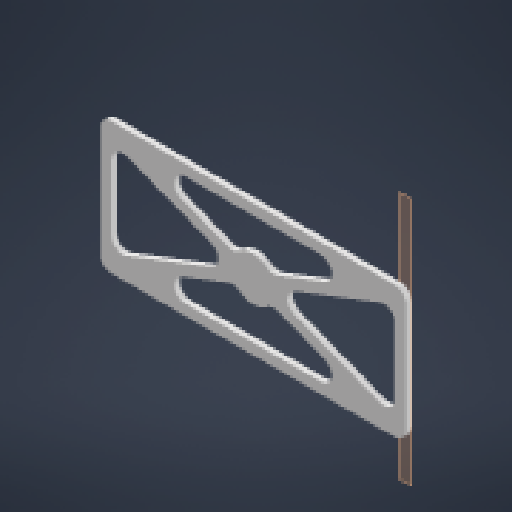
# Autodesk Inventor part: bracing
Saved by Autodesk Inventor 2026.3 (Build 303398000, 398)
## iProperties
Created: 2026-05-06
Part Number: bracing
Material: Generic
Document SubType Name: Modeling
Designer: frede
Density: 1 g/cm^3
Appearance: Default
Author: frede
Autodesk Inventor part; units mm, degrees
ref_plane "YZ Plane" through (0, 0, 0) normal (1, 0, 0) x (0, 1, 0)
ref_plane "XZ Plane" through (0, 0, 0) normal (0, 1, 0) x (-1, 0, 0)
ref_plane "XY Plane" through (0, 0, 0) normal (0, 0, 1) x (1, 0, 0)
ref_plane "Work Plane1" through (0, 0, 0) normal (0, 0, 1) x (1, 0, 0)
sketch "Sketch1" plane through (0, 0, 0) normal (0, 0, 1) x (1, 0, 0)
  line L0 (5, -30) -> (5, -90)
  line L1 (-134, -30) -> (-134, -90)
  line L2 (5, -90) -> (-134, -90)
  line L3 (-134, -30) -> (5, -30)
  line L4 (5, 0) -> (5, -102.9406) projected
  line L5 (0, -35) -> (-129, -35)
  line L6 (-129, -35) -> (-129, -85)
  line L7 (-129, -85) -> (0, -85)
  line L8 (0, -85) -> (0, -35)
  line L9 (0, -35) -> (-129, -85)
  line L10 (0, -85) -> (-129, -35)
  circle A0 centre (-64.5, -60) radius 10
  circle A1 centre (-64.5, -60) radius 2.5
  line L11 (0, -82.3188) -> (-122.0824, -35)
  line L12 (-6.9176, -85) -> (-129, -37.6812)
  line L13 (-122.0824, -85) -> (0, -37.6812)
  line L14 (-129, -82.3188) -> (-6.9176, -35)
  point P0 (0, 0)
  point P1 (-43.2477, -65.5561)
  point P2 (-40.0223, -72.1687)
  point P3 (-54.5685, -58.8318)
  point P4 (0, -17.9417)
  point P5 (-54.5685, -61.1682)
  point P6 (-74.4315, -58.8318)
  point P7 (-72.6245, -54.1697)
  point P8 (-72.6245, -65.8303)
  point P9 (-56.3755, -65.8303)
  point P10 (-57.5824, -60)
  point P11 (-74.4315, -61.1682)
  point P12 (-56.3755, -54.1697)
  dimension "d0" = 60
  dimension "d1" = 139
  dimension "d2" = 0
  dimension "d3" = 50
  dimension "d4" = 129
  dimension "d5" = 5
  dimension "d6" = 5
  dimension "d7" = 20
  dimension "d8" = 5
  dimension "d14" = 30
  constraints: 28 end point, 10 point on line, 8 parallel, 4 tangent, 2 centre point, 2 horizontal, 1 coincident, 1 midpoint, 1 perpendicular
  measures "d0" distance between parallel lines of L3 L2
  measures "d1" distance between parallel lines of L1 L0
  measures "d2" distance between parallel lines of L4 L0
  measures "d3" distance of L6.end L5.end
  measures "d4" distance between parallel lines of L6 L8
  measures "d5" distance between parallel lines of L2 L7
  measures "d6" distance between parallel lines of L0 L8
  measures "d7" diameter of A0
  measures "d8" diameter of A1
  measures "d14" distance from line of point (0, 0) L3
extrude "Extrusion1" add sketch "Sketch1" along normal blind 2.5 contours L0 L2 L1 L3 | L9 A0 L14 L5 | L8 L13 A0 L9 | A0 L13 L11 L9 | L9 L11 L14 A0 | L11 A0 L10 L5 | L14 L11 A0 | L8 L10 A0 L11 | A0 L11 L13 | L11 L13 L10 A1 L9 | L9 A1 L11 | L10 A0 L12 L6 | L11 L14 L10 A0 | L11 A1 L14 | L7 L12 A0 L10 | A0 L10 L13 L11 | A1 L10 L9 | L9 L10 A1 | L10 L14 L12 A0 | A1 L10 L14 | A0 L12 L13 L10 | L13 A1 L10 | L10 A1 L9 | L9 A1 L10 | L14 A0 L9 L6 | L12 L14 A0 | L10 A1 L9 L12 L14 | L7 L9 A0 L13 | A0 L13 L12 | L13 L12 A1 | A1 L12 L9 | L14 L12 L9 A0 | A0 L9 L12 L13
fillet "Fillet1" radius 5 20 edges at (-6.9176, -85, 1.25) (0, -82.3188, 1.25) (-122.0824, -85, 1.25) (-129, -82.3188, 1.25) (-129, -37.6812, 1.25) (-122.0824, -35, 1.25) (-6.9176, -35, 1.25) (0, -37.6812, 1.25) (-54.5685, -61.1682, 1.25) (-56.3755, -65.8303, 1.25) (-72.6245, -65.8303, 1.25) (-74.4315, -61.1682, 1.25) (-74.4315, -58.8318, 1.25) (-72.6245, -54.1697, 1.25) (-56.3755, -54.1697, 1.25) (5, -90, 1.25) (-134, -90, 1.25) (-134, -30, 1.25) (5, -30, 1.25) (-54.5685, -58.8318, 1.25)
equation "\"d5\" = -0.5 * d3 + 0.5 * d0"
equation "\"d6\" = -0.5 * d4 + 0.5 * d1"
body "Solid1"
